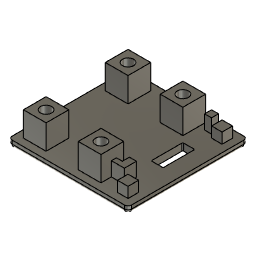
airbee_bottom (Autodesk Fusion 360 design; units mm, degrees)
Autodesk Fusion 360 part; units mm, degrees
sketch "Skizze1" plane through (0, 0, 0) normal (0, 0, 1) x (1, 0, 0)
  line L0 (-14.9, 14.9) -> (14.9, 14.9)
  line L1 (14.9, 14.9) -> (14.9, -14.9)
  line L2 (14.9, -14.9) -> (-14.9, -14.9)
  line L3 (-14.9, -14.9) -> (-14.9, 14.9)
  line L4 (9.15, -2.3) -> (12.05, -2.3)
  line L5 (12.3, -2.05) -> (12.3, 6.45)
  line L6 (12.05, 6.7) -> (9.15, 6.7)
  line L7 (8.9, 6.45) -> (8.9, -2.05)
  arc A0 (8.9, -2.05) -> (9.15, -2.3) centre (9.15, -2.05) ccw
  arc A1 (9.15, 6.7) -> (8.9, 6.45) centre (9.15, 6.45) ccw
  arc A2 (12.3, 6.45) -> (12.05, 6.7) centre (12.05, 6.45) ccw
  arc A3 (12.05, -2.3) -> (12.3, -2.05) centre (12.05, -2.05) ccw
  line L8 (-17, 17) -> (17, 17)
  line L9 (17, 17) -> (17, -17)
  line L10 (17, -17) -> (-17, -17)
  line L11 (-17, -17) -> (-17, 17)
  point P0 (8.9, -2.3)
  point P1 (12.3, -2.3)
  point P2 (8.9, 6.7)
  dimension "d1" = 14.9
  dimension "d3" = 14.9
  dimension "d4" = 29.8
  dimension "d161" = 3.4
  dimension "d162" = 9
  dimension "d164" = 2.6
  dimension "d165" = 0.25
  dimension "d189" = 8.2
  dimension "d190" = -2.1
  constraint horizontal L0
  constraint vertical L1
  constraint horizontal L2
  constraint vertical L3
  constraint horizontal L4
  constraint vertical L5
  constraint horizontal L6
  constraint vertical L7
  constraint coincident P0 L4
  constraint coincident P0 L7
  constraint tangent L4 A0
  constraint tangent L7 A0
  constraint coincident P2 L7
  constraint coincident P2 L6
  constraint tangent L7 A1
  constraint tangent L6 A1
  constraint equal A0 A1
  constraint tangent L5 A2
  constraint tangent L6 A2
  constraint equal A0 A2
  constraint coincident P1 L4
  constraint coincident P1 L5
  constraint tangent L4 A3
  constraint tangent L5 A3
  constraint equal A0 A3
  constraint equal L0 L3
  measures "d1" distance of origin L1
  measures "d3" distance of origin L2
  measures "d4" distance of L0.start L2.end
  measures "d161" distance of P0 P1
  measures "d162" distance of P0 P2
  measures "d164" distance of L1 L5
  measures "d165" radius of A0
  measures "d189" distance of L0 L6
extrude "Extrusion12" add sketch "Skizze1" along normal blind 2 contours L0 L1 L2 L3 | L8 L9 L10 L11
sketch "Skizze4" plane through (0, 0, 2) normal (0, 0, 1) x (-1, 0, 0)
  circle A0 centre (3.85, 0) radius 9.6
  line L0 (14.9, -14.9) -> (-14.9, -14.9)
  circle A1 centre (3.85, 0) radius 11.6
  line L1 (14.9, -14.9) -> (8.4346, -14.9)
  line L2 (8.4346, -14.9) -> (8.4346, -8.4346)
  line L3 (8.4346, -8.4346) -> (14.9, -8.4346)
  line L4 (14.9, -8.4346) -> (14.9, -14.9)
  line L5 (14.9, 14.9) -> (8.4346, 14.9)
  line L6 (8.4346, 14.9) -> (8.4346, 8.4346)
  line L7 (8.4346, 8.4346) -> (14.9, 8.4346)
  line L8 (14.9, 8.4346) -> (14.9, 14.9)
  line L9 (-7.2, -10.4) -> (-7.2, 15)
  line L10 (-0.7346, -14.9) -> (-7.2, -14.9)
  line L11 (-7.2, -14.9) -> (-7.2, -8.4346)
  line L12 (-7.2, -8.4346) -> (-0.7346, -8.4346)
  line L13 (-0.7346, -8.4346) -> (-0.7346, -14.9)
  line L14 (-0.7346, 14.9) -> (-7.2, 14.9)
  line L15 (-7.2, 14.9) -> (-7.2, 8.4346)
  line L16 (-7.2, 8.4346) -> (-0.7346, 8.4346)
  line L17 (-0.7346, 8.4346) -> (-0.7346, 14.9)
  line L18 (-14.9, -14.9) -> (-14.9, 14.9)
  arc A2 (-12.05, 2.3) -> (-12.3, 2.05) centre (-12.05, 2.05) ccw
  line L19 (-12.05, 2.3) -> (-9.15, 2.3)
  arc A3 (-8.9, 2.05) -> (-9.15, 2.3) centre (-9.15, 2.05) ccw
  line L20 (-8.9, 2.05) -> (-8.9, -6.45)
  arc A4 (-9.15, -6.7) -> (-8.9, -6.45) centre (-9.15, -6.45) ccw
  line L21 (-9.15, -6.7) -> (-12.05, -6.7)
  arc A5 (-12.3, -6.45) -> (-12.05, -6.7) centre (-12.05, -6.45) ccw
  line L22 (-12.3, -6.45) -> (-12.3, 2.05)
  line L23 (-7.2, -14.9) -> (-8.9, -14.9)
  line L24 (-8.9, -14.9) -> (-8.9, 10.5)
  line L25 (-8.9, 10.5) -> (-7.2, 10.5)
  line L26 (-7.2, 10.5) -> (-7.2, -14.9)
  line L27 (-7.2, 11.9417) -> (-10.9, 11.9417)
  line L28 (-10.9, 11.9417) -> (-10.9, 12.5)
  line L29 (-10.9, 12.5) -> (-7.2, 12.5)
  line L30 (-7.2, 12.5) -> (-7.2, 11.9417)
  line L31 (-10.9, 11.9417) -> (-10.9, 8.5)
  line L32 (-10.8993, -14.9) -> (-10.9, -12.9)
  line L33 (-10.9, -12.9) -> (-8.9, -12.9)
  line L34 (-10.9, 8.5) -> (-8.9, 8.5)
  line L35 (17, 17) -> (-17, 17)
  line L36 (-17, 17) -> (-17, -17)
  line L37 (-17, -17) -> (17, -17)
  line L38 (17, -17) -> (17, 17)
  line L39 (8.4346, 14.9) -> (-0.7346, 14.9)
  line L40 (8.4346, -14.9) -> (-0.7346, -14.9)
  line L41 (14.9, -8.4346) -> (14.9, 8.4346)
  line L42 (3.85, 0) -> (14.9, -3.18)
  line L43 (3.85, 0) -> (14.9, 3.18)
  line L44 (-0.7346, 8.4346) -> (-7.2, 14.9)
  line L45 (-7.2, 8.4346) -> (-0.7346, 14.9)
  line L46 (14.9, 14.9) -> (8.4346, 8.4346)
  line L47 (8.4346, 14.9) -> (14.9, 8.4346)
  line L48 (8.4346, -8.4346) -> (14.9, -14.9)
  line L49 (8.4346, -14.9) -> (14.9, -8.4346)
  line L50 (-7.2, -8.4346) -> (-0.7346, -14.9)
  line L51 (-7.2, -14.9) -> (-0.7346, -8.4346)
  line L52 (-14.9, 14.9) -> (-11.9, 14.9)
  line L53 (-11.9, 14.9) -> (-11.9, 11.9)
  line L54 (-11.9, 11.9) -> (-14.9, 11.9)
  line L55 (-14.9, 11.9) -> (-14.9, 14.9)
  line L56 (-14.9, -14.9) -> (-11.9, -14.9)
  line L57 (-11.9, -14.9) -> (-11.9, -11.9)
  line L58 (-11.9, -11.9) -> (-14.9, -11.9)
  line L59 (-14.9, -11.9) -> (-14.9, -14.9)
  point P0 (-3.9673, -11.6673)
  point P1 (11.6673, -11.6673)
  point P2 (11.6673, 11.6673)
  point P3 (-3.9673, 11.6673)
  dimension "d134" = 19.2
  dimension "d135" = 14.9
  dimension "d136" = 2
  dimension "d178" = 1.7
  dimension "d179" = 25.4
  dimension "d181" = 3.7
  dimension "d182" = 2
  dimension "d183" = 2
  dimension "d184" = 2
  dimension "d185" = 6
  dimension "d188" = 2
  dimension "d194" = 2.1
  dimension "d195" = 2.1
  dimension "d196" = 2.1
  dimension "d197" = 4
  dimension "d214" = 3
  dimension "d215" = 3
  dimension "d216" = 3
  dimension "d217" = 3
  constraint horizontal L1
  constraint vertical L2
  constraint horizontal L3
  constraint vertical L4
  constraint coincident L0.start L1.start
  constraint horizontal L5
  constraint vertical L6
  constraint horizontal L7
  constraint vertical L8
  constraint vertical L9
  constraint horizontal L10
  constraint vertical L11
  constraint horizontal L12
  constraint vertical L13
  constraint coincident L9 L11.end
  constraint coincident L0 L10.start
  constraint horizontal L14
  constraint vertical L15
  constraint horizontal L16
  constraint vertical L17
  constraint coincident L9 L15.end
  constraint coincident A0 L6.end
  constraint coincident A0 L16.end
  constraint coincident A0 L12.end
  constraint coincident A0 L2.end
  constraint horizontal L23
  constraint vertical L24
  constraint horizontal L25
  constraint vertical L26
  constraint horizontal L27
  constraint vertical L28
  constraint horizontal L29
  constraint vertical L30
  constraint coincident L9 L27.start
  constraint perpendicular L19 L31
  constraint coincident L0 L32.start
  constraint coincident L24 L33.end
  constraint perpendicular L24 L33
  constraint perpendicular L24 L34
  constraint equal L5 L14
  constraint equal L6 L7
  constraint equal L16 L17
  constraint equal L2 L3
  constraint equal L12 L13
  constraint coincident A0.centre A1.centre
  constraint coincident L41 L42.end
  constraint coincident L41 L43.end
  constraint midpoint L50 P0
  constraint midpoint L49 P1
  constraint midpoint L46 P2
  constraint midpoint L45 P3
  constraint horizontal L52
  constraint vertical L53
  constraint horizontal L54
  constraint vertical L55
  constraint coincident L18.end L52.start
  constraint horizontal L56
  constraint vertical L57
  constraint horizontal L58
  constraint vertical L59
  constraint coincident L0.end L18.start
  measures "d134" diameter of A0
  measures "d135" distance of A0.centre L0
  measures "d178" distance of L10.end L23.end
  measures "d179" distance of L10.end L25.end
  measures "d181" distance of L28.end L29.end
  measures "d182" distance of L32.start L32.end
  measures "d183" distance of L32.end L33.end
  measures "d184" distance of L31.end L34.end
  measures "d185" distance of L18 L24
  measures "d188" distance of L25 L29
  measures "d194" distance of L5 L35
  measures "d195" distance of L14 L35
  measures "d196" distance of L8 L38
  measures "d197" distance of L29 L34
  measures "d214" distance of L18.end L52.end
  measures "d215" distance of L18.end L54.end
  measures "d216" distance of L0.end L56.end
  measures "d217" distance of L0.end L58.end
extrude "Extrusion17" add sketch "Skizze4" along normal blind 7 contours A1 L7 L46 | A1 L6 L46 | A1 L17 L44 | A1 L16 L44 | A1 L6 L46 L47 | A1 L7 L46 L47 | A1 L12 L51 | A1 L13 L51 | A1 L16 L44 L45 | A1 L17 L44 L45 | L5 L46 L47 | L8 L46 L47 | A1 L2 L48 | A1 L3 L48 | A1 L12 L50 L51 | A1 L13 L50 L51 | L9 L15 L26 L30 L44 L45 | L14 L44 L45 | A1 L2 L48 L49 | A1 L3 L48 L49 | L9 L11 L26 L50 L51 | L0 L10 L50 L51 | L0 L1 L48 L49 | L4 L48 L49
extrude "Extrusion20" add sketch "Skizze4" along normal blind 4 contours L9 L15 L24 L25 L27 L31 L34 | L0 L24 L32 L33
fillet "Abrundung1" radius 1 8 edges at (17, 0, 0) (0, 17, 0) (-17, 0, 0) (0, -17, 0) (17, -17, 1) (-17, -17, 1) (-17, 17, 1) (17, 17, 1)
sketch "Skizze10" plane through (0, 0, 0) normal (0, 0, -1) x (1, 0, 0)
  arc A0 (12.3, 2.05) -> (12.05, 2.3) centre (12.05, 2.05) ccw
  line L0 (12.3, 2.05) -> (12.3, -6.45)
  arc A1 (12.05, -6.7) -> (12.3, -6.45) centre (12.05, -6.45) ccw
  line L1 (12.05, -6.7) -> (9.15, -6.7)
  arc A2 (8.9, -6.45) -> (9.15, -6.7) centre (9.15, -6.45) ccw
  line L2 (8.9, -6.45) -> (8.9, 2.05)
  arc A3 (9.15, 2.3) -> (8.9, 2.05) centre (9.15, 2.05) ccw
  line L3 (9.15, 2.3) -> (12.05, 2.3)
  line L4 (16, 16) -> (-16, 16)
  line L5 (-16, 16) -> (-16, -16)
  line L6 (-16, -16) -> (16, -16)
  line L7 (16, -16) -> (16, 16)
  line L8 (14.9, -14.9) -> (-14.9, -14.9)
  line L9 (-14.9, -14.9) -> (-14.9, 14.9)
  line L10 (-14.9, 14.9) -> (14.9, 14.9)
  line L11 (14.9, 14.9) -> (14.9, -14.9)
  line L12 (14.9, -14.9) -> (7.2, -14.9)
  line L13 (7.2, -14.9) -> (7.2, 14.9)
  line L14 (7.2, 14.9) -> (14.9, 14.9)
  line L15 (14.9, 14.9) -> (14.9, -14.9)
  line L16 (7.2, 14.9) -> (0.7346, 14.9)
  line L17 (0.7346, 14.9) -> (0.7346, 8.4346)
  line L18 (0.7346, 8.4346) -> (7.2, 8.4346)
  line L19 (7.2, 8.4346) -> (7.2, 14.9)
  line L20 (-14.9, 14.9) -> (-8.4346, 14.9)
  line L21 (-8.4346, 14.9) -> (-8.4346, 8.4346)
  line L22 (-8.4346, 8.4346) -> (-14.9, 8.4346)
  line L23 (-14.9, 8.4346) -> (-14.9, 14.9)
  line L24 (-14.9, -14.9) -> (-8.4346, -14.9)
  line L25 (-8.4346, -14.9) -> (-8.4346, -8.4346)
  line L26 (-8.4346, -8.4346) -> (-14.9, -8.4346)
  line L27 (-14.9, -8.4346) -> (-14.9, -14.9)
  line L28 (7.2, -14.9) -> (0.7346, -14.9)
  line L29 (0.7346, -14.9) -> (0.7346, -8.4346)
  line L30 (0.7346, -8.4346) -> (7.2, -8.4346)
  line L31 (7.2, -8.4346) -> (7.2, -14.9)
  circle A4 centre (-3.85, 0) radius 9.6
  line L32 (14.9, 14.9) -> (11.9, 14.9)
  line L33 (11.9, 14.9) -> (11.9, 11.9)
  line L34 (11.9, 11.9) -> (14.9, 11.9)
  line L35 (14.9, 11.9) -> (14.9, 14.9)
  line L36 (14.9, -14.9) -> (11.9, -14.9)
  line L37 (11.9, -14.9) -> (11.9, -11.9)
  line L38 (11.9, -11.9) -> (14.9, -11.9)
  line L39 (14.9, -11.9) -> (14.9, -14.9)
  point P0 (3.9673, 11.6673)
  point P1 (-11.6673, 11.6673)
  point P2 (-11.6673, -11.6673)
  point P3 (3.9673, -11.6673)
  dimension "d200" = 1.1
  dimension "d201" = 1.1
  dimension "d202" = 1.1
  dimension "d203" = 1.1
  dimension "d204" = 7.7
  dimension "d205" = 19.2
  dimension "d210" = 3
  dimension "d211" = 3
  dimension "d212" = 3
  dimension "d213" = 3
  constraint horizontal L8
  constraint vertical L9
  constraint horizontal L10
  constraint vertical L11
  constraint horizontal L12
  constraint vertical L13
  constraint horizontal L14
  constraint vertical L15
  constraint coincident L10 L13.end
  constraint horizontal L16
  constraint vertical L17
  constraint horizontal L18
  constraint vertical L19
  constraint horizontal L20
  constraint vertical L21
  constraint horizontal L22
  constraint vertical L23
  constraint horizontal L24
  constraint vertical L25
  constraint horizontal L26
  constraint vertical L27
  constraint horizontal L28
  constraint vertical L29
  constraint horizontal L30
  constraint vertical L31
  constraint coincident L29.end A4
  constraint coincident L25.end A4
  constraint coincident L21.end A4
  constraint coincident L17.end A4
  constraint equal L29 L30
  constraint equal L25 L26
  constraint equal L25 L29
  constraint equal L17 L18
  constraint equal L21 L22
  constraint equal L18 L30
  constraint horizontal L32
  constraint vertical L33
  constraint horizontal L34
  constraint vertical L35
  constraint horizontal L36
  constraint vertical L37
  constraint horizontal L38
  constraint vertical L39
  measures "d200" distance of L5 L9
  measures "d201" distance of L4 L10
  measures "d202" distance of L7 L11
  measures "d203" distance of L6 L8
  measures "d204" distance of L11 L13
  measures "d205" diameter of A4
  measures "d210" distance of L10.end L32.end
  measures "d211" distance of L10.end L34.end
  measures "d212" distance of L8.start L36.end
  measures "d213" distance of L8.start L38.end
hole "Bohrung4" at (3.9673, 11.6673, 0) at (-11.6673, 11.6673, 0) at (3.9673, -11.6673, 0) at (-11.6673, -11.6673, 0) direction (0, 0, 1) diameter 3.2 end up to surface (9 mm away) countersink diameter 6 countersink angle 90
extrude "Extrusion21" add sketch "Skizze4" along normal blind 3 contours L0 L18 L56 L57 L58 L59 | L18 L52 L53 L54 L55
equation "d1 = ( 29.8 / 2 ) * 1 mm"
equation "d3 = ( 29.8 / 2 ) * 1 mm"
equation "d135 = ( 29.8 / 2 ) * 1 mm"
equation "d164 = 6 mm - 3.4 mm"
equation "d181 = 1.7 mm + 2 mm"
equation "d189 = ( 25.4 / 2 ) * 1 mm - 4.5 mm"
